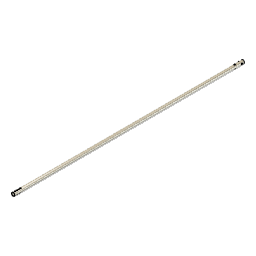
0.885.6603 - Tube 28 (longueur=1.900m) - IGTE 21484_232257 Rep. 104 (Autodesk Fusion 360 design; units mm, degrees)
Autodesk Fusion 360 part; units mm, degrees
sketch "Sketch1" plane through (0, 0, 0) normal (0, 0, 1) x (1, 0, 0)
  circle A0 centre (0, 0) radius 14
  circle A1 centre (0, 0) radius 10.9
  dimension "d1" = 28
  dimension "d2" = 3.1
  constraint coincident A0.centre A1.centre
  measures "d1" diameter of A0
extrude "Extrude1" add sketch "Sketch1" along normal blind 1900
sketch "Sketch2" plane through (0, 0, 0) normal (0, 1, 0) x (1, 0, 0)
  line L0 (0, 0) -> (0, -68) construction
  circle A0 centre (0, -68) radius 6
  line L1 (-14, -1900) -> (14, -1900)
  line L2 (0, -1900) -> (0, -1885) construction
  circle A1 centre (0, -1885) radius 4.5
  circle A2 centre (0, -1870) radius 4.5
  circle A3 centre (0, -1855) radius 4.5
  circle A4 centre (0, -1840) radius 4.5
  dimension "d5" = 68
  dimension "d6" = 12
  dimension "d7" = 15
  dimension "d8" = 9
  dimension "d11" = 15
  dimension "d12" = 26
  constraint coincident L0.start origin
  constraint coincident L0.end A0.centre
  constraint midpoint L1 L2.start
  constraint coincident L2.end A1.centre
  measures "d5" distance of L0.start L0.end
  measures "d6" diameter of A0
  measures "d7" distance of L2.start L2.end
  measures "d8" diameter of A1
extrude "Extrude2" cut sketch "Sketch2" along normal through all and the other way through all
sketch "Sketch3" plane through (0, 0, 0) normal (1, 0, 0) x (0, 0, -1)
  line L0 (0, 0) -> (-20, 0) construction
  circle A0 centre (-20, 0) radius 6
  dimension "d15" = 20
  dimension "d16" = 12
  constraint coincident L0.start origin
  constraint coincident L0.end A0.centre
  measures "d15" distance of L0.start L0.end
  measures "d16" diameter of A0
extrude "Extrude3" cut sketch "Sketch3" along normal through all and the other way through all
